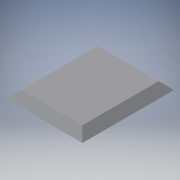
# Autodesk Inventor part: hologram display base (for assembly)
Saved by Autodesk Inventor 2016 (Build 200138000, 138)
## iProperties
Created: 2017-10-23
Part Number: hologram display base (for assembly)
Material: Generic
Document SubType Name: Modeling
Designer: student
Density: 1 g/cm^3
Appearance: Default
Author: student
Autodesk Inventor part; units mm, degrees
ref_plane "YZ Plane" through (0, 0, 0) normal (1, 0, 0) x (0, 1, 0)
ref_plane "XZ Plane" through (0, 0, 0) normal (0, 1, 0) x (-1, 0, 0)
ref_plane "XY Plane" through (0, 0, 0) normal (0, 0, 1) x (1, 0, 0)
sketch "Sketch1" plane through (0, 0, 0) normal (0, 1, 0) x (-1, 0, 0)
  line L0 (-254, 304.8) -> (254, 304.8)
  line L1 (254, 304.8) -> (254, -304.8)
  line L2 (254, -304.8) -> (-254, -304.8)
  line L3 (-254, -304.8) -> (-254, 304.8)
  line L4 (-254, 304.8) -> (254, -304.8) construction
  line L5 (254, 304.8) -> (-254, -304.8) construction
  point P0 (0, 0)
  dimension "d0" = 609.6
  dimension "d1" = 508
  constraints: 12 end point, 2 midpoint, 2 parallel, 1 horizontal, 1 perpendicular
  measures "d0" distance of L0.end L1.end
  measures "d1" distance of L1.end L2.end
extrude "Extrusion1" add sketch "Sketch1" along normal blind 50.8
chamfer "Chamfer1" distance 50.8 angle 45 4 edges at (254, 50.8, 0) (0, 50.8, -304.8) (-254, 50.8, 0) (0, 50.8, 304.8)
body "Solid1"
